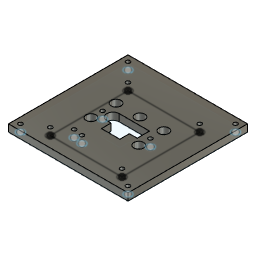
InnerCube-Top (Autodesk Fusion 360 design; units mm, degrees)
Autodesk Fusion 360 part; units mm, degrees
note: some values were not read from the file. Set by a fixed rule: which sketch regions a step uses.
sketch "Skizze1" plane through (0, 0, 0) normal (0, 0, 1) x (1, 0, 0)
  line L0 (0, 0) -> (100, 0)
  line L1 (100, 0) -> (100, 100)
  line L2 (100, 100) -> (0, 100)
  line L3 (0, 100) -> (0, 0)
  circle A0 centre (50, 48.75) radius 2.2909
  line L4 (38.8, 53.75) -> (64.2, 53.75)
  line L5 (64.2, 53.75) -> (64.2, 43.45)
  line L6 (64.2, 43.45) -> (38.8, 43.45)
  line L7 (38.8, 43.45) -> (38.8, 53.75)
  circle A1 centre (38.8, 48.6) radius 5.15
  line L8 (42.3, 43.45) -> (57.7, 43.45)
  line L9 (57.7, 43.45) -> (57.7, 35.45)
  line L10 (57.7, 35.45) -> (42.3, 35.45)
  line L11 (42.3, 35.45) -> (42.3, 43.45)
  dimension "d1" = 100
  dimension "d2" = 100
  dimension "d5" = 50
  dimension "d6" = 48.75
  dimension "d7" = 10.3
  dimension "d8" = 25.4
  dimension "d9" = 6.5
  dimension "d10" = 15.4
  dimension "d11" = 5
  dimension "d12" = 14.2
  dimension "d13" = 8
  constraint horizontal L0
  constraint vertical L1
  constraint horizontal L2
  constraint vertical L3
  constraint coincident L0.start L3.end
  constraint horizontal L4
  constraint vertical L5
  constraint horizontal L6
  constraint vertical L7
  constraint midpoint L7 A1.centre
  constraint coincident L4.start A1
  constraint horizontal L8
  constraint vertical L9
  constraint horizontal L10
  constraint vertical L11
  constraint coincident L6 L8.start
  measures "d1" distance of L0.start L0.end
  measures "d2" distance of L0.start L2.end
  measures "d5" distance of L3 A0.centre
  measures "d6" distance of L0 A0.centre
  measures "d7" distance of L4.end L5.end
  measures "d8" distance of L4.start L4.end
  measures "d9" distance of L5 L9
  measures "d10" distance of L9.end L10.end
  measures "d11" distance of A0.centre L4
  measures "d12" distance of A0.centre L5
  measures "d13" distance of L8.start L10.end
extrude "Extrusion1" add sketch "Skizze1" along normal blind 6 contours L0 L1 L2 L3
sketch "Skizze4" plane through (0, 0, 6) normal (0, 0, 1) x (-1, 0, 0)
  arc A0 (-38.8, -53.75) -> (-38.8, -43.45) centre (-38.8, -48.6) ccw
  line L0 (-38.8, -53.75) -> (-64.2, -53.75)
  line L1 (-64.2, -53.75) -> (-64.2, -43.45)
  line L2 (-64.2, -43.45) -> (-57.7, -43.45)
  line L3 (-57.7, -43.45) -> (-57.7, -35.45)
  line L4 (-57.7, -35.45) -> (-42.3, -35.45)
  line L5 (-42.3, -35.45) -> (-42.3, -43.45)
  line L6 (-42.3, -43.45) -> (-38.8, -43.45)
  line L7 (0, -100) -> (0, 0)
  line L8 (0, 0) -> (-100, 0)
  line L9 (-100, 0) -> (-100, -100)
  line L10 (-100, -100) -> (0, -100)
  line L11 (-57.7, -35.45) -> (-50, -35.45)
  line L12 (-50, -35.45) -> (-50, -26.45)
  line L13 (-50, -26.45) -> (-57.7, -26.45)
  line L14 (-57.7, -26.45) -> (-57.7, -35.45)
  line L15 (-50, -26.45) -> (-31.5, -26.45)
  line L16 (-31.5, -26.45) -> (-31.5, -23.45)
  line L17 (-31.5, -23.45) -> (-50, -23.45)
  line L18 (-50, -23.45) -> (-50, -26.45)
  line L19 (-50, -23.45) -> (-39, -23.45)
  line L20 (-39, -23.45) -> (-39, -22.45)
  line L21 (-39, -22.45) -> (-50, -22.45)
  line L22 (-50, -22.45) -> (-50, -23.45)
  circle A1 centre (-31.5, -23.45) radius 1.7
  circle A2 centre (-39, -22.45) radius 1.7
  circle A3 centre (-95, -5) radius 1.7
  circle A4 centre (-5, -5) radius 1.7
  circle A5 centre (-5, -95) radius 1.7
  circle A6 centre (-95, -95) radius 1.7
  circle A7 centre (-30, -48.75) radius 1.7
  circle A8 centre (-70, -48.75) radius 1.7
  dimension "d14" = 7.7
  dimension "d15" = 9
  dimension "d16" = 18.5
  dimension "d17" = 3
  dimension "d18" = 11
  dimension "d19" = 1
  dimension "d20" = 3.4
  dimension "d21" = 3.4
  dimension "d28" = 3.4
  dimension "d29" = 3.4
  dimension "d30" = 3.4
  dimension "d31" = 3.4
  dimension "d32" = 5
  dimension "d33" = 5
  dimension "d34" = 5
  dimension "d35" = 5
  dimension "d36" = 5
  dimension "d37" = 5
  dimension "d38" = 5
  dimension "d39" = 5
  dimension "d46" = 3.4
  dimension "d47" = 3.4
  dimension "d48" = 48.75
  dimension "d49" = 48.75
  dimension "d50" = 40
  dimension "d51" = 30
  constraint horizontal L11
  constraint vertical L12
  constraint horizontal L13
  constraint vertical L14
  constraint coincident L3.end L4.start
  constraint horizontal L15
  constraint vertical L16
  constraint horizontal L17
  constraint vertical L18
  constraint horizontal L19
  constraint vertical L20
  constraint horizontal L21
  constraint vertical L22
  constraint coincident L16.end L17.start
  constraint coincident L20.end L21.start
  measures "d14" distance of L3.end L11.end
  measures "d15" distance of L3.end L13.end
  measures "d16" distance of L12.end L15.end
  measures "d17" distance of L12.end L17.end
  measures "d18" distance of L17.end L19.end
  measures "d19" distance of L17.end L21.end
  measures "d20" diameter of A1
  measures "d21" diameter of A2
  measures "d28" diameter of A3
  measures "d29" diameter of A4
  measures "d30" diameter of A5
  measures "d31" diameter of A6
  measures "d32" distance of L10 A5.centre
  measures "d33" distance of L7 A5.centre
  measures "d34" distance of L9 A6.centre
  measures "d35" distance of L10 A6.centre
  measures "d36" distance of L8 A3.centre
  measures "d37" distance of L9 A3.centre
  measures "d38" distance of L7 A4.centre
  measures "d39" distance of L8 A4.centre
  measures "d46" diameter of A7
  measures "d47" diameter of A8
  measures "d48" distance of L8 A7.centre
  measures "d49" distance of L8 A8.centre
  measures "d50" distance of A7.centre A8.centre
  measures "d51" distance of L7 A7.centre
extrude "Extrusion2" cut sketch "Skizze4" against normal blind 5 contours L16 L17 A1 | L16 L17 A1 | L17 L19 L20 L21 A2 | L17 L19 A2 | L17 L20 L21 A2 | A3 | A4 | A5 | A6 | A7 | A8
sketch "Skizze5" plane through (0, 0, 0) normal (0, 0, -1) x (1, 0, 0)
  arc A0 (38.8, -43.45) -> (38.8, -53.75) centre (38.8, -48.6) ccw
  line L0 (38.8, -43.45) -> (42.3, -43.45)
  line L1 (42.3, -43.45) -> (42.3, -35.45)
  line L2 (42.3, -35.45) -> (57.7, -35.45)
  line L3 (57.7, -35.45) -> (57.7, -43.45)
  line L4 (57.7, -43.45) -> (64.2, -43.45)
  line L5 (64.2, -43.45) -> (64.2, -53.75)
  line L6 (64.2, -53.75) -> (38.8, -53.75)
  line L7 (0, 0) -> (0, -100)
  line L8 (0, -100) -> (100, -100)
  line L9 (100, -100) -> (100, 0)
  line L10 (100, 0) -> (0, 0)
  circle A1 centre (39, -22.45) radius 3
  circle A2 centre (31.5, -23.45) radius 3
  circle A3 centre (30, -48.75) radius 3
  circle A4 centre (70, -48.75) radius 3
  circle A5 centre (95, -95) radius 3
  circle A6 centre (5, -95) radius 3
  circle A7 centre (5, -5) radius 3
  circle A8 centre (95, -5) radius 3
  line L11 (20, -15) -> (80, -15)
  line L12 (80, -15) -> (80, -80)
  line L13 (80, -80) -> (20, -80)
  line L14 (20, -80) -> (20, -15)
  circle A9 centre (20, -15) radius 3
  circle A10 centre (80, -15) radius 3
  circle A11 centre (80, -80) radius 3
  circle A12 centre (20, -80) radius 3
  circle A13 centre (20, -15) radius 1.7
  circle A14 centre (80, -15) radius 1.7
  circle A15 centre (20, -80) radius 1.7
  circle A16 centre (80, -80) radius 1.7
  dimension "d24" = 6
  dimension "d25" = 6
  dimension "d56" = 6
  dimension "d57" = 6
  dimension "d58" = 6
  dimension "d59" = 6
  dimension "d60" = 6
  dimension "d61" = 6
  dimension "d81" = 20
  dimension "d82" = 20
  dimension "d83" = 15
  dimension "d84" = 60
  dimension "d85" = 20
  dimension "d86" = 6
  dimension "d87" = 6
  dimension "d88" = 6
  dimension "d89" = 6
  dimension "d90" = 3.4
  dimension "d91" = 3.4
  dimension "d92" = 3.4
  dimension "d95" = 3.4
  constraint horizontal L11
  constraint vertical L12
  constraint horizontal L13
  constraint vertical L14
  constraint coincident L11.start L14.end
  constraint coincident L11.end L12.start
  constraint coincident L12.end L13.start
  constraint coincident L13.end L14.start
  constraint concentric A9 A13
  constraint concentric A10 A14
  constraint concentric A12 A15
  constraint concentric A11 A16
  measures "d24" diameter of A1
  measures "d25" diameter of A2
  measures "d56" diameter of A3
  measures "d57" diameter of A4
  measures "d58" diameter of A5
  measures "d59" diameter of A6
  measures "d60" diameter of A7
  measures "d61" diameter of A8
  measures "d81" distance of L7 L14
  measures "d82" distance of L9 L12
  measures "d83" distance of L10 L11
  measures "d84" distance of L12.end L13.end
  measures "d85" distance of L8 L13
  measures "d86" diameter of A9
  measures "d87" diameter of A10
  measures "d88" diameter of A11
  measures "d89" diameter of A12
  measures "d90" diameter of A13
  measures "d91" diameter of A14
  measures "d92" diameter of A15
  measures "d95" diameter of A16
extrude "Extrusion3" cut sketch "Skizze5" against normal blind 2.5 contours A1 | A2 | A3 | A4 | A5 | A6 | A7 | A8 | L11 L14 A13 | L11 L14 A13 | L11 L14 A9 A13 | L11 L14 A9 A13 | L11 L12 A10 A14 | L11 L12 A10 A14 | L13 L14 A12 A15 | L13 L14 A12 A15 | L11 L12 A14 | L11 L12 A14 | L13 L14 A15 | L13 L14 A15 | L12 L13 A11 A16 | L12 L13 A11 A16 | L12 L13 A16 | L12 L13 A16
sketch "Skizze8" plane through (0, 0, 6) normal (0, 0, 1) x (-1, 0, 0)
  circle A0 centre (-5, -95) radius 1.7
  circle A1 centre (-39, -22.45) radius 1.7
  circle A2 centre (-5, -5) radius 1.7
  circle A3 centre (-30, -48.75) radius 1.7
  circle A4 centre (-95, -95) radius 1.7
  circle A5 centre (-31.5, -23.45) radius 1.7
  circle A6 centre (-95, -5) radius 1.7
  circle A7 centre (-70, -48.75) radius 1.7
  arc A8 (-38.8, -53.75) -> (-38.8, -43.45) centre (-38.8, -48.6) ccw
  line L0 (-38.8, -53.75) -> (-64.2, -53.75)
  line L1 (-64.2, -53.75) -> (-64.2, -43.45)
  line L2 (-64.2, -43.45) -> (-57.7, -43.45)
  line L3 (-57.7, -43.45) -> (-57.7, -35.45)
  line L4 (-57.7, -35.45) -> (-42.3, -35.45)
  line L5 (-42.3, -35.45) -> (-42.3, -43.45)
  line L6 (-42.3, -43.45) -> (-38.8, -43.45)
  line L7 (0, -100) -> (0, 0)
  line L8 (0, 0) -> (-100, 0)
  line L9 (-100, 0) -> (-100, -100)
  line L10 (-100, -100) -> (0, -100)
  circle A9 centre (-30, -60) radius 4.1
  circle A10 centre (-70, -60) radius 4.1
  circle A11 centre (-70, -39) radius 4.1
  circle A12 centre (-30, -39) radius 4.1
  circle A13 centre (-50, -60) radius 4.1
  dimension "d62" = 8.2
  dimension "d63" = 40
  dimension "d64" = 40
  dimension "d65" = 40
  dimension "d66" = 50
  dimension "d67" = 30
  dimension "d68" = 30
  dimension "d69" = 30
  dimension "d70" = 30
  dimension "d71" = 39
  dimension "d72" = 39
  constraint equal A9 A13
  constraint equal A10 A13
  constraint equal A10 A11
  constraint equal A11 A12
  measures "d62" diameter of A9
  measures "d63" distance of L10 A9.centre
  measures "d64" distance of L10 A13.centre
  measures "d65" distance of L10 A10.centre
  measures "d66" distance of L9 A13.centre
  measures "d67" distance of L9 A10.centre
  measures "d68" distance of L7 A9.centre
  measures "d69" distance of L7 A12.centre
  measures "d70" distance of L9 A11.centre
  measures "d71" distance of L8 A11.centre
  measures "d72" distance of L8 A12.centre
extrude "Extrusion5" cut sketch "Skizze8" against normal blind 5.5 contours A9 | A10 | A11 | A12 | A13
extrude "Extrusion7" cut sketch "Skizze5" against normal blind 6 contours L11 L14 A13 | L11 L14 A13 | L11 L12 A14 | L11 L12 A14 | L13 L14 A15 | L13 L14 A15 | L12 L13 A16 | L12 L13 A16
sketch "Skizze9" plane through (0, 0, 6) normal (0, 0, 1) x (-1, 0, 0)
  circle A0 centre (-70, -60) radius 4.1
  circle A1 centre (-50, -60) radius 4.1
  circle A2 centre (-70, -39) radius 4.1
  circle A3 centre (-30, -60) radius 4.1
  circle A4 centre (-30, -39) radius 4.1
  circle A5 centre (-5, -95) radius 1.7
  circle A6 centre (-39, -22.45) radius 1.7
  circle A7 centre (-5, -5) radius 1.7
  circle A8 centre (-30, -48.75) radius 1.7
  circle A9 centre (-95, -95) radius 1.7
  circle A10 centre (-31.5, -23.45) radius 1.7
  circle A11 centre (-95, -5) radius 1.7
  circle A12 centre (-70, -48.75) radius 1.7
  arc A13 (-38.8, -53.75) -> (-38.8, -43.45) centre (-38.8, -48.6) ccw
  line L0 (-38.8, -53.75) -> (-64.2, -53.75)
  line L1 (-64.2, -53.75) -> (-64.2, -43.45)
  line L2 (-64.2, -43.45) -> (-57.7, -43.45)
  line L3 (-57.7, -43.45) -> (-57.7, -35.45)
  line L4 (-57.7, -35.45) -> (-42.3, -35.45)
  line L5 (-42.3, -35.45) -> (-42.3, -43.45)
  line L6 (-42.3, -43.45) -> (-38.8, -43.45)
  line L7 (0, -100) -> (0, 0)
  line L8 (0, 0) -> (-100, 0)
  line L9 (-100, 0) -> (-100, -100)
  line L10 (-100, -100) -> (0, -100)
  line L11 (0, -100) -> (-100, -100)
  line L12 (-100, -100) -> (-100, 0)
  line L13 (-100, 0) -> (0, 0)
  line L14 (0, 0) -> (0, -100)
  line L15 (-8, -92) -> (-92, -92)
  line L16 (-92, -92) -> (-92, -8)
  line L17 (-92, -8) -> (-8, -8)
  line L18 (-8, -8) -> (-8, -92)
  dimension "d75" = 8
  dimension "d76" = 8
  dimension "d77" = 8
  dimension "d78" = 8
  constraint horizontal L11
  constraint vertical L12
  constraint horizontal L13
  constraint vertical L14
  constraint coincident L8.end L9.start
  constraint coincident L7.start L10.end
  constraint horizontal L15
  constraint vertical L16
  constraint horizontal L17
  constraint vertical L18
  measures "d75" distance of L14 L18
  measures "d76" distance of L11 L15
  measures "d77" distance of L13 L17
  measures "d78" distance of L12 L16
extrude "Extrusion6" [rolled back] along distance -6 taper angle 0
equation "d14 = 15.400 mm / 2"
equation "d16 = 23 mm - 4.5 mm"
equation "d18 = 23 mm - 12 mm"
